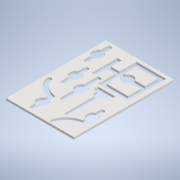
# Autodesk Inventor part: PiezaACortarApoyoInicialV3_0
Saved by Autodesk Inventor 2021 (Build 250183000, 183)
## iProperties
Created: 2022-11-08
Part Number: PiezaACortarApoyoInicialV3_0
Material: Genérico
Document SubType Name: Modeling
Designer: ivanm
Density: 1 g/cm^3
Appearance: Valor por defecto
Author: ivanm
Autodesk Inventor part; units mm, degrees
ref_plane "YZ Plane" through (0, 0, 0) normal (1, 0, 0) x (0, 1, 0)
ref_plane "XZ Plane" through (0, 0, 0) normal (0, 1, 0) x (-1, 0, 0)
ref_plane "XY Plane" through (0, 0, 0) normal (0, 0, 1) x (1, 0, 0)
sketch "Boceto1" plane through (0, 0, 0) normal (0, 1, 0) x (-1, 0, 0)
  line L0 (-351.1493, 111.6779) -> (-31.1493, 111.6779) projected
  line L1 (-351.1493, -358.3221) -> (-351.1493, 111.6779) projected
  line L2 (-31.1493, -358.3221) -> (-351.1493, -358.3221) projected
  line L3 (-31.1493, 111.6779) -> (-31.1493, -358.3221) projected
  line L4 (-91.4425, -195.3008) -> (-91.4425, -165.7136) projected
  arc A0 (-111.4425, -195.3008) -> (-91.4425, -195.3008) centre (-101.4425, -195.3008) ccw projected
  line L5 (-111.4425, -165.7136) -> (-111.4425, -195.3008) projected
  arc A1 (-111.4425, -119.8879) -> (-111.4425, -165.7136) centre (-101.4425, -142.8008) ccw projected
  line L6 (-111.4425, -90.3008) -> (-111.4425, -119.8879) projected
  arc A2 (-91.4425, -90.3008) -> (-111.4425, -90.3008) centre (-101.4425, -90.3008) ccw projected
  line L7 (-91.4425, -119.8879) -> (-91.4425, -90.3008) projected
  arc A3 (-91.4425, -165.7136) -> (-91.4425, -119.8879) centre (-101.4425, -142.8008) ccw projected
  circle A4 centre (-101.4425, -90.3008) radius 4 projected
  circle A5 centre (-101.4425, -195.3008) radius 4 projected
  line L8 (-57.9631, -335.3262) -> (-57.9631, -305.739) projected
  arc A6 (-77.9631, -335.3262) -> (-57.9631, -335.3262) centre (-67.9631, -335.3262) ccw projected
  line L9 (-77.9631, -305.739) -> (-77.9631, -335.3262) projected
  arc A7 (-77.9631, -259.9133) -> (-77.9631, -305.739) centre (-67.9631, -282.8262) ccw projected
  line L10 (-77.9631, -230.3262) -> (-77.9631, -259.9133) projected
  arc A8 (-57.9631, -230.3262) -> (-77.9631, -230.3262) centre (-67.9631, -230.3262) ccw projected
  line L11 (-57.9631, -259.9133) -> (-57.9631, -230.3262) projected
  arc A9 (-57.9631, -305.739) -> (-57.9631, -259.9133) centre (-67.9631, -282.8262) ccw projected
  circle A10 centre (-67.9631, -230.3262) radius 4 projected
  circle A11 centre (-67.9631, -335.3262) radius 4 projected
  circle A12 centre (-320.1388, -332.8331) radius 4 projected
  circle A13 centre (-320.1388, -172.8331) radius 4 projected
  line L12 (-150.1388, -312.8331) -> (-130.1388, -312.8331) projected
  line L13 (-150.1388, -262.8331) -> (-150.1388, -312.8331) projected
  line L14 (-190.1388, -262.8331) -> (-150.1388, -262.8331) projected
  line L15 (-190.1388, -342.8331) -> (-190.1388, -262.8331) projected
  line L16 (-330.1388, -342.8331) -> (-190.1388, -342.8331) projected
  line L17 (-330.1388, -162.8331) -> (-330.1388, -342.8331) projected
  line L18 (-190.1388, -162.8331) -> (-330.1388, -162.8331) projected
  line L19 (-190.1388, -242.8331) -> (-190.1388, -162.8331) projected
  line L20 (-150.1388, -242.8331) -> (-190.1388, -242.8331) projected
  line L21 (-150.1388, -192.8331) -> (-150.1388, -242.8331) projected
  line L22 (-130.1388, -192.8331) -> (-150.1388, -192.8331) projected
  line L23 (-130.1388, -312.8331) -> (-130.1388, -192.8331) projected
  circle A14 centre (-140.1388, -303.8331) radius 4 projected
  circle A15 centre (-140.1388, -201.8331) radius 4 projected
  line L24 (-210.1388, -262.8331) -> (-210.1388, -322.8331) projected
  line L25 (-216.2259, -262.8331) -> (-210.1388, -262.8331) projected
  arc A16 (-262.0517, -262.8331) -> (-216.2259, -262.8331) centre (-239.1388, -252.8331) ccw projected
  line L26 (-310.1388, -262.8331) -> (-262.0517, -262.8331) projected
  line L27 (-310.1388, -322.8331) -> (-310.1388, -262.8331) projected
  line L28 (-210.1388, -322.8331) -> (-310.1388, -322.8331) projected
  line L29 (-210.1388, -242.8331) -> (-216.2259, -242.8331) projected
  line L30 (-210.1388, -182.8331) -> (-210.1388, -242.8331) projected
  line L31 (-310.1388, -182.8331) -> (-210.1388, -182.8331) projected
  line L32 (-310.1388, -242.8331) -> (-310.1388, -182.8331) projected
  line L33 (-262.0517, -242.8331) -> (-310.1388, -242.8331) projected
  arc A17 (-216.2259, -242.8331) -> (-262.0517, -242.8331) centre (-239.1388, -252.8331) ccw projected
  line L34 (-265.9681, -131.0427) -> (-281.4732, -131.0427) projected
  arc A18 (-251.4732, -103.1298) -> (-265.9681, -131.0427) centre (-241.4732, -126.0427) ccw projected
  line L35 (-251.4732, 38.9573) -> (-251.4732, -103.1298) projected
  line L36 (-231.4732, 38.9573) -> (-251.4732, 38.9573) projected
  line L37 (-231.4732, -103.1298) -> (-231.4732, 38.9573) projected
  arc A19 (-216.9783, -131.0427) -> (-231.4732, -103.1298) centre (-241.4732, -126.0427) ccw projected
  line L38 (-201.4732, -131.0427) -> (-216.9783, -131.0427) projected
  line L39 (-201.4732, -151.0427) -> (-201.4732, -131.0427) projected
  line L40 (-281.4732, -151.0427) -> (-201.4732, -151.0427) projected
  line L41 (-281.4732, -131.0427) -> (-281.4732, -151.0427) projected
  circle A20 centre (-207.4732, -141.0427) radius 4 projected
  circle A21 centre (-275.4732, -141.0427) radius 4 projected
  circle A22 centre (-168.8154, -182.57) radius 4 projected
  line L42 (-178.8154, -12.57) -> (-178.8154, -79.6571) projected
  line L43 (-158.8154, -12.57) -> (-178.8154, -12.57) projected
  line L44 (-158.8154, -79.6571) -> (-158.8154, -12.57) projected
  arc A23 (-158.8154, -125.4828) -> (-158.8154, -79.6571) centre (-168.8154, -102.57) ccw projected
  line L45 (-158.8154, -192.57) -> (-158.8154, -125.4828) projected
  line L46 (-178.8154, -192.57) -> (-158.8154, -192.57) projected
  line L47 (-178.8154, -125.4828) -> (-178.8154, -192.57) projected
  arc A24 (-178.8154, -79.6571) -> (-178.8154, -125.4828) centre (-168.8154, -102.57) ccw projected
  circle A25 centre (-168.8154, -22.57) radius 4 projected
  line L48 (-141.4407, -2.8264) -> (-141.4407, 19.2607) projected
  arc A26 (-141.4407, 65.0864) -> (-141.4407, 19.2607) centre (-131.4407, 42.1736) ccw projected
  line L49 (-141.4407, 65.0864) -> (-141.4407, 87.1736) projected
  arc A27 (-121.4407, 87.1736) -> (-141.4407, 87.1736) centre (-131.4407, 87.1736) ccw projected
  line L50 (-121.4407, 87.1736) -> (-121.4407, 65.0864) projected
  arc A28 (-121.4407, 19.2607) -> (-121.4407, 65.0864) centre (-131.4407, 42.1736) ccw projected
  line L51 (-121.4407, 19.2607) -> (-121.4407, 5.729) projected
  arc A29 (-45.2358, -64.3067) -> (-121.4407, 5.729) centre (-141.2403, -92.2913) ccw projected
  arc A30 (-64.4367, -69.9037) -> (-45.2358, -64.3067) centre (-54.8362, -67.1052) ccw projected
  arc A31 (-64.4367, -69.9037) -> (-132.5295, -12.767) centre (-141.2403, -92.2913) ccw projected
  arc A32 (-141.4407, -2.8264) -> (-132.5295, -12.767) centre (-131.4407, -2.8264) ccw projected
  circle A33 centre (-131.4407, 87.1736) radius 4 projected
  circle A34 centre (-131.4407, -2.8264) radius 4 projected
  line L52 (-321.9456, 30.3713) -> (-321.9456, 8.2841) projected
  arc A35 (-313.0345, 40.3118) -> (-321.9456, 30.3713) centre (-311.9456, 30.3713) ccw projected
  arc A36 (-313.0345, 40.3118) -> (-244.9416, 97.4485) centre (-321.7452, 119.8362) ccw projected
  arc A37 (-225.7407, 91.8516) -> (-244.9416, 97.4485) centre (-235.3412, 94.65) ccw projected
  arc A38 (-301.9456, 21.8159) -> (-225.7407, 91.8516) centre (-321.7452, 119.8362) ccw projected
  line L53 (-301.9456, 8.2841) -> (-301.9456, 21.8159) projected
  arc A39 (-301.9456, -37.5416) -> (-301.9456, 8.2841) centre (-311.9456, -14.6287) ccw projected
  line L54 (-301.9456, -59.6287) -> (-301.9456, -37.5416) projected
  arc A40 (-321.9456, -59.6287) -> (-301.9456, -59.6287) centre (-311.9456, -59.6287) ccw projected
  line L55 (-321.9456, -37.5416) -> (-321.9456, -59.6287) projected
  arc A41 (-321.9456, 8.2841) -> (-321.9456, -37.5416) centre (-311.9456, -14.6287) ccw projected
  circle A42 centre (-311.9456, -59.6287) radius 4 projected
  circle A43 centre (-311.9456, 30.3713) radius 4 projected
  point P0 (0, 0)
extrude "Extrusión1" add sketch "Boceto1" along normal blind 10 contours L0 L3 L2 L1 | L24 L28 L27 L26 A16 L25 | L29 A17 L33 L32 L31 L30
